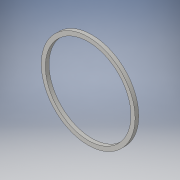
# Autodesk Inventor part: RTS  o-ring
Saved by Autodesk Inventor 2016 (Build 200138000, 138)
## iProperties
Created: 2016-10-07
Part Number: RTS  o-ring
Material: Generic
Document SubType Name: Modeling
Designer: sullir
Density: 1 g/cm^3
Appearance: Default
Author: sullir
Autodesk Inventor part; units mm, degrees
ref_plane "YZ Plane" through (0, 0, 0) normal (1, 0, 0) x (0, 1, 0)
ref_plane "XZ Plane" through (0, 0, 0) normal (0, 1, 0) x (-1, 0, 0)
ref_plane "XY Plane" through (0, 0, 0) normal (0, 0, 1) x (1, 0, 0)
sketch "Sketch1" plane through (0, 0, 0) normal (0, 0, 1) x (1, 0, 0)
  circle A0 centre (0, 0) radius 32.387
  constraints: 1 centre point, 1 coincident
extrude "Extrusion1" add sketch "Sketch1" along normal blind 2.54
sketch "Sketch2" plane through (0, 0, 0) normal (0, 0, -1) x (-1, 0, 0)
  circle A0 centre (0, 0) radius 29.3964
  constraints: 1 centre point, 1 coincident
hole "Hole1" at (0, 0, 0) at (0, 0, 0) direction (0, 0, 1) diameter 59.055 end through all
body "Solid1"
